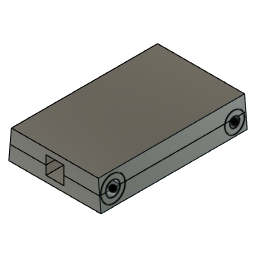
Wing to mainrod connector v6 (Autodesk Fusion 360 design; units mm, degrees)
Autodesk Fusion 360 part; units mm, degrees
sketch "Main cross-section sketch" plane through (0, 0, 0) normal (0, 1, 0) x (1, 0, 0)
  line L0 (6.1, -6.1) -> (-6.1, -6.1)
  line L1 (-6.1, -6.1) -> (-6.1, 6.1)
  line L2 (-6.1, 6.1) -> (6.1, 6.1)
  line L3 (6.1, 6.1) -> (6.1, -6.1)
  line L4 (29.75, -10.1) -> (-29.75, -10.1)
  line L5 (-29.75, -10.1) -> (-31.5173, 10.1)
  line L6 (-31.5173, 10.1) -> (31.5173, 10.1)
  line L7 (31.5173, 10.1) -> (29.75, -10.1)
  line L8 (-29.75, -10.1) -> (29.75, -10.1)
  line L9 (-6.1, -6.1) -> (-30.1, -6.1) construction
  line L10 (6.1, -6.1) -> (30.1, -6.1) construction
  line L11 (6.1, -6.1) -> (-6.1, 6.1) construction
  line L12 (6.1, 6.1) -> (-6.1, -6.1) construction
  dimension "d13" = 85
  dimension "d14" = 85
  dimension "d20" = 24
  dimension "d22" = 4
  dimension "d25" = 4
  dimension "d26" = 12.2
  constraint equal L1 L2
  constraint horizontal L8
  constraint horizontal L0
  constraint equal L0 L1
  constraint coincident L5 L9.end
  constraint vertical L1
  constraint horizontal L9
  constraint vertical L3
  constraint equal L0 L3
  constraint coincident L7 L10.end
  constraint parallel L0 L10
  constraint equal L9 L10
  constraint midpoint L11 origin
  measures "d13" angle of L5 L6
  measures "d14" angle of L6 L7
  measures "d20" distance of L0.end L9.end
  measures "d22" distance of L0 L4
  measures "d25" distance of L2 L6
  measures "d26" distance of L0.start L2.end
extrude "Extrude1" add sketch "Main cross-section sketch" along normal blind 100 makes body 1
sketch "Right side sketch" plane through (30.401, 0, 2.6597) normal (0.996195, 0, 0.087156) x (0, 1, 0)
  line L0 (0, 7.4687) -> (0, -12.8085)
  line L1 (0, -12.8085) -> (100, -12.8085)
  line L2 (100, -12.8085) -> (100, 7.4687)
  line L3 (100, 7.4687) -> (0, 7.4687)
  circle A0 centre (9, -2.6699) radius 4.825
  circle A1 centre (92.0226, -4.7633) radius 3.24
  line L4 (9, -2.6699) -> (0, -2.6699) construction
  line L5 (9, -2.6699) -> (92.0226, -2.6699) construction
  line L6 (92.0226, -2.6699) -> (100, -2.6699) construction
  circle A2 centre (9, -2.6699) radius 8.275
  circle A3 centre (92.0226, -4.7633) radius 6.69
  dimension "d31" = 9.65
  dimension "d32" = 6.48
  dimension "d35" = 16.55
  dimension "d36" = 13.38
  dimension "d44" = 9
  dimension "d64" = 2.0934
  dimension "d65" = 83.0226
  constraint midpoint L0 L4.end
  constraint coincident A0.centre L4.start
  constraint parallel L4 L5
  constraint midpoint L2 L6.end
  constraint perpendicular L2 L6
  constraint parallel L5 L6
  constraint concentric A0 A2
  constraint concentric A1 A3
  measures "d31" diameter of A0
  measures "d32" diameter of A1
  measures "d35" diameter of A2
  measures "d36" diameter of A3
  measures "d44" distance of L0 A0.centre
  measures "d64" distance of A1.centre L5
  measures "d65" horizontal distance of A1.centre A0.centre
extrude "Extrude5" add sketch "Right side sketch" along normal blind 20 contours A2 | A3 bodies 1
mirror "Mirror1" about plane through (0, 0, 0) normal (1, 0, 0) of 6 faces at (37.3468, 17.2339, -0.2398) (50.6143, 16.0762, 1.0948) (43.9372, 13.819, 0.9225) (44.1278, 98.7043, -1.2555) (50.783, 97.5257, -0.8337) (43.8413, 90.6901, 2.0187) on bodies 1
extrude "Extrude6" add sketch "Right side sketch" along normal blind 20 contours L0 L1 L2 L3 bodies 1
extrude "Extrude7" add 1 faces at (-30.0108, 67.572, 7.1192) along direction (-0.996195, 0, 0.087156) blind 20 on bodies 1 bodies 1
split "Split1" by plane through (0, 0, 0) normal (0, 0, 1) bodies 1 makes body 2 at (9.9167, 33.3333, 10.1)
move_body "Move1" bodies 2 to x (-1, 0, 0) y (0, 1, 0) z (0, 0, -1) at (62.2, 0, 0.2)
delete_body "RemoveBody1" bodies 1
delete_body "RemoveBody2" bodies 2
extrude "Extrude8" add sketch "Main cross-section sketch" along normal blind 100 separate body makes body 3
extrude "Extrude9" cut sketch "Right side sketch" against normal blind 20 contours A0 | A1 bodies 3
mirror "Mirror2" about plane through (0, 0, 0) normal (1, 0, 0) of "Extrude9"
split "Split2" by plane through (0, 0, 0) normal (0, 0, 1) bodies 3 makes body 4 at (9.9167, 33.3333, 10.1)
extrude "Extrude4" [rolled back] along distance 20 taper angle 0
extrude "Extrude2" [rolled back] along distance 10 taper angle 0
sketch "Left side sketch" plane through (-11.8041, 0, 1.0327) normal (-0.996195, 0, 0.087156) x (0, -1, 0)
  line L0 (0, -9.9817) -> (0, 8.2879)
  line L1 (0, 8.2879) -> (-100, 8.2879)
  line L2 (-100, 8.2879) -> (-100, -9.9817)
  line L3 (-100, -9.9817) -> (0, -9.9817)
  circle A0 centre (-92.0226, -2.9403) radius 5.19
  circle A1 centre (-92.0226, -2.9403) radius 3.19
  circle A2 centre (-9, -0.8469) radius 4.775
  circle A3 centre (-9, -0.8469) radius 6.775
  line L4 (-100, -0.8469) -> (0, -0.8469) construction
  dimension "d40" = 9.55
  dimension "d41" = 6.38
  dimension "d42" = 13.55
  dimension "d43" = 10.38
  dimension "d47" = 9
  dimension "d66" = 2.0934
  dimension "d67" = 83.0226
  constraint concentric A2 A3
  constraint concentric A0 A1
  constraint midpoint L2 L4.start
  constraint midpoint L0 L4.end
  constraint coincident A2.centre L4
  measures "d40" diameter of A2
  measures "d41" diameter of A1
  measures "d42" diameter of A3
  measures "d43" diameter of A0
  measures "d47" distance of L0 A2.centre
  measures "d66" distance of A0.centre L4
  measures "d67" horizontal distance of A2.centre A0.centre
extrude "Extrude3" [rolled back] along distance 10 taper angle 0
hole "Hole1" [rolled back] hole depth 12 hole diameter 3.1 tip angle 180
hole "Hole2" [rolled back] hole depth 12 hole diameter 3.1 tip angle 180
hole "Hole3" [rolled back] hole depth 18 hole diameter 3.1 tip angle 180
hole "Hole4" [rolled back] hole depth 18 hole diameter 3.1 tip angle 180
equation "d35 = 9.55 mm + 7 mm"
equation "d36 = 6.38 mm + 7 mm"
equation "d42 = 9.55 mm + 4 mm"
equation "d43 = 6.38 mm + 4 mm"
